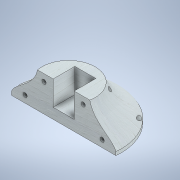
# Autodesk Inventor part: Podstawa 01-2
Saved by Autodesk Inventor 2021 (Build 250183000, 183)
## iProperties
Created: 2021-11-03
Part Number: Podstawa 01-2
Material: Generic
Document SubType Name: Modeling
Designer: Łukasz
Density: 1 g/cm^3
Appearance: Wood - Painted White
Author: Łukasz
Autodesk Inventor part; units mm, degrees
ref_plane "YZ Plane" through (0, 0, 0) normal (1, 0, 0) x (0, 1, 0)
ref_plane "XZ Plane" through (0, 0, 0) normal (0, 1, 0) x (-1, 0, 0)
ref_plane "XY Plane" through (0, 0, 0) normal (0, 0, 1) x (1, 0, 0)
sketch "Sketch1" plane through (0, 0, 0) normal (0, 0, 1) x (1, 0, 0)
  line L0 (0, 0) -> (-75, 0)
  line L1 (0, 0) -> (0, 50)
  line L2 (0, 50) -> (-38, 50)
  line L3 (-75, 0) -> (-75, 5)
  spline S0 degree 3 poles (-38, 50) (-46.7224, 6.6996) (-125.1064, 18.5226) (-28.5296, -55.0422) knots 0 0 0 0 1 1 1 1
  point P0 (-58.1914, 22.009)
  dimension "d0" = 75
  dimension "d1" = 50
  dimension "d2" = 38
  dimension "d3" = 5
  constraints: 8 end point, 2 horizontal, 2 vertical, 4 other
  measures "d0" distance of L0.start L0.end
  measures "d1" distance of L0.start L1.end
  measures "d2" distance of L1.end L2.end
  measures "d3" distance of L0.end L3.end
revolve "Revolution1" add sketch "Sketch1" angle 360 about axis through (0, 0, 0) along (0, 1, 0)
sketch "Sketch2" plane through (0, 50, 0) normal (0, 1, 0) x (1, 0, 0)
  line L0 (-15, 24) -> (15, 24)
  line L1 (15, 24) -> (15, -24)
  line L2 (15, -24) -> (-15, -24)
  line L3 (-15, -24) -> (-15, 24)
  point P0 (0, 0)
  dimension "d5" = 30
  dimension "d6" = 48
  dimension "d7" = 24
  dimension "d8" = 15
  constraints: 8 end point, 2 parallel, 1 horizontal, 1 perpendicular
  measures "d5" distance of L1.end L2.end
  measures "d6" distance of L0.end L1.end
  measures "d7" distance from line of point (0, 0) L0
  measures "d8" distance from line of L3 point (0, 0)
extrude "Extrusion1" cut sketch "Sketch2" against normal blind 35
sketch "Sketch3" plane through (0, 15, 0) normal (0, 1, 0) x (1, 0, 0)
  line L0 (15, -24) -> (-15, -24) projected
  line L1 (-15, -24) -> (-15, 24) projected
  line L2 (15, -24) -> (-15, -24)
  line L3 (-15, -24) -> (-15, -7)
  line L4 (-15, -7) -> (15, -7)
  line L5 (15, -7) -> (15, -24)
  point P0 (0, 0)
  dimension "d11" = 17
  constraints: 8 end point, 2 parallel, 1 horizontal, 1 perpendicular, 1 point on line
  measures "d11" distance of L2.end L3.end
extrude "Extrusion2" cut sketch "Sketch3" against normal blind 8
sketch "Sketch4" plane through (0, 0, 0) normal (0, 0, 1) x (1, 0, 0)
  circle A0 centre (-28, 40) radius 3
  circle A1 centre (-55, 10) radius 3
  line L0 (75, 0) -> (-75, 0) projected
  line L1 (38, 50) -> (-38, 50) projected
  line L2 (-75, 0) -> (-75, 5) projected
  line L3 (15, 50) -> (-15, 50) construction
  line L4 (0, 50) -> (0, 20.8019) construction
  circle A2 centre (28, 40) radius 3
  circle A3 centre (55, 10) radius 3
  point P0 (0, 0)
  dimension "d14" = 6
  dimension "d15" = 6
  dimension "d16" = 10
  dimension "d17" = 10
  dimension "d18" = 20
  dimension "d19" = 10
  constraints: 4 centre point, 2 end point, 2 symmetric about line, 1 midpoint, 1 vertical, 2 other
  measures "d14" diameter of A0
  measures "d15" diameter of A1
  measures "d16" distance from line of L0 A1.centre
  measures "d17" distance from line of L1 A0.centre
  measures "d18" distance from line of L2 A1.centre
  measures "d19" horizontal distance of L1.end A0.centre
extrude "Extrusion3" cut sketch "Sketch4" along normal blind 52 and the other way blind 52
ref_plane "Work Plane1" through (-15, 15, 7) normal (0, 0, 1) x (1, 0, 0)
split "Split1" plane through (-15, 15, 7) removes the side toward (0, 0, 1)
equation "\"d7\" = 0.5 * d6"
equation "\"d8\" = 0.5 * d5"
body "Solid1"
